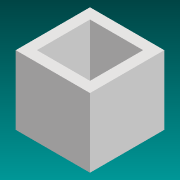
# Autodesk Inventor part: 龙门架柱1
Saved by Autodesk Inventor 2021 (Build 250183000, 183)
## iProperties
Created: 2025-04-17
Part Number: 龙门架柱1
Material: 常规
Document SubType Name: Modeling
Designer: 86155
Density: 1 g/cm^3
Appearance: 默认
Author: 86155
Autodesk Inventor part; units mm, degrees
ref_plane "YZ Plane" through (0, 0, 0) normal (1, 0, 0) x (0, 1, 0)
ref_plane "XY Plane" through (0, 0, 0) normal (0, 0, 1) x (1, 0, 0)
sketch "草图1" plane through (0, 0, 0) normal (0, 1, 0) x (-1, 0, 0)
  line L0 (0, 0) -> (-70, 0)
  line L1 (-70, 0) -> (-70, -70)
  line L2 (-70, -70) -> (0, -70)
  line L3 (0, -70) -> (0, 0)
  dimension "d0" = 70
  dimension "d1" = 70
  constraints: 8 end point, 2 parallel, 1 horizontal, 1 perpendicular
  measures "d0" distance of L2.end L1.end
  measures "d1" distance of L1.end L0.end
extrude "拉伸1" add sketch "草图1" along normal blind 5
sketch "草图2" plane through (0, 5, 0) normal (0, 1, 0) x (1, 0, 0)
  line L0 (0, 70) -> (0, 0) projected
  line L1 (70, 70) -> (0, 70) projected
  line L2 (0, 0) -> (70, 0)
  line L3 (70, 0) -> (70, 70)
  line L4 (70, 70) -> (0, 70)
  line L5 (0, 70) -> (0, 0)
  line L6 (60, 60) -> (60, 10)
  line L7 (60, 10) -> (10, 10)
  line L8 (10, 10) -> (10, 60)
  line L9 (10, 60) -> (60, 60)
  dimension "d4" = 10
  constraints: 16 end point, 4 parallel, 2 perpendicular, 1 horizontal, 3 other
  measures "d4" distance between parallel lines of L3 L6
extrude "拉伸2" add sketch "草图2" along normal blind 60
fillet "圆角1" radius 5 8 edges at (0, 32.5, 0) (35, 0, 0) (0, 0, -35) (35, 0, -70) (70, 0, -35) (70, 32.5, -70) (70, 32.5, 0) (0, 32.5, -70)
sketch "草图3" plane through (0, 65, 0) normal (0, 1, 0) x (1, 0, 0)
  arc A0 (0, 5) -> (5, 0) centre (5, 5) ccw projected
  line L0 (5, 0) -> (65, 0) projected
  arc A1 (65, 0) -> (70, 5) centre (65, 5) ccw projected
  line L1 (70, 5) -> (70, 65) projected
  arc A2 (70, 65) -> (65, 70) centre (65, 65) ccw projected
  line L2 (65, 70) -> (5, 70) projected
  arc A3 (5, 70) -> (0, 65) centre (5, 65) ccw projected
  line L3 (0, 65) -> (0, 5) projected
  line L4 (60, 60) -> (60, 10) projected
  line L5 (60, 10) -> (10, 10) projected
  line L6 (10, 10) -> (10, 60) projected
  line L7 (10, 60) -> (60, 60) projected
  line L8 (68.5, 65) -> (68.5, 5)
  arc A4 (65, 1.5) -> (68.5, 5) centre (65, 5) ccw
  line L9 (65, 1.5) -> (5, 1.5)
  arc A5 (1.5, 5) -> (5, 1.5) centre (5, 5) ccw
  line L10 (1.5, 5) -> (1.5, 65)
  arc A6 (5, 68.5) -> (1.5, 65) centre (5, 65) ccw
  line L11 (5, 68.5) -> (65, 68.5)
  arc A7 (68.5, 65) -> (65, 68.5) centre (65, 65) ccw
  line L12 (1.5, 45) -> (0, 45)
  line L13 (0, 65) -> (0, 5) projected
  line L14 (1.5, 25) -> (0, 25)
  point P0 (0, 0)
  dimension "d8" = 1.5
  dimension "d9" = 25
  dimension "d10" = 25
  constraints: 12 end point, 8 point on circle, 4 centre point, 4 point on line, 2 perpendicular, 7 other
  measures "d8" distance between parallel lines of L1 L8
  measures "d9" distance between parallel lines of L2 L12
  measures "d10" distance between parallel lines of L0 L14
extrude "拉伸3" add sketch "草图3" along normal blind 450 contours L3 L14 L10 A5 L9 A4 L8 A7 L11 A6 L12 A3 L2 A2 L1 A1 L0 A0
ref_plane "工作平面1" through (0, 130, 0) normal (0, 1, 0) x (-1, 0, 0)
sketch "草图5" plane through (0, 130, 0) normal (0, 1, 0) x (-1, 0, 0)
  arc A0 (-70, -65) -> (-65, -70) centre (-65, -65) ccw projected
  line L0 (-65, -70) -> (-5, -70)
  line L1 (-5, -70) -> (-5, -80)
  line L2 (-5, -80) -> (-65, -80)
  line L3 (-65, -80) -> (-65, -70)
  point P0 (0, 0)
  dimension "d18" = 10
  constraints: 8 end point, 2 parallel, 1 horizontal, 1 perpendicular
  measures "d18" distance of L0.end L1.end
extrude "拉伸4" add sketch "草图5" along normal blind 10
fillet "圆角2" radius 10 2 edges at (65, 135, -80) (5, 135, -80)
sketch "草图6" plane through (0, 140, 0) normal (0, 1, 0) x (1, 0, 0)
  point P0 (0, 0)
sketch "草图7" plane through (0, 140, 0) normal (0, 1, 0) x (1, 0, 0)
  arc A0 (65, 70) -> (55, 80) centre (55, 70) ccw projected
  line L0 (55, 80) -> (15, 80) projected
  arc A1 (15, 80) -> (5, 70) centre (15, 70) ccw projected
  arc A2 (62.5, 70) -> (55, 77.5) centre (55, 70) ccw
  line L1 (55, 77.5) -> (15, 77.5)
  arc A3 (15, 77.5) -> (7.5, 70) centre (15, 70) ccw
  line L2 (62.5, 70) -> (7.5, 70)
  line L3 (60, 10) -> (60, 60) projected
  point P0 (0, 0)
  dimension "d22" = 2.5
  constraints: 4 end point, 4 point on circle, 2 centre point, 1 perpendicular, 2 other
  measures "d22" radial gap between concentric circles of A0 A2
extrude "拉伸5" cut sketch "草图7" against normal blind 2
ref_plane "工作平面2" through (0, 485, 0) normal (0, 1, 0) x (1, 0, 0)
sketch "草图8" plane through (0, 485, 0) normal (0, 1, 0) x (1, 0, 0)
  arc A0 (15, 80) -> (5, 70) centre (15, 70) ccw projected
  line L0 (55, 80) -> (15, 80) projected
  arc A1 (65, 70) -> (55, 80) centre (55, 70) ccw projected
  line L1 (5, 70) -> (65, 70) projected
  point P0 (0, 0)
extrude "拉伸6" add sketch "草图8" along normal blind 10
sketch "草图9" plane through (0, 485, 0) normal (0, -1, 0) x (1, 0, 0)
  line L0 (15, -77.5) -> (55, -77.5) projected
  arc A0 (7.5, -70) -> (15, -77.5) centre (15, -70) ccw projected
  line L1 (62.5, -70) -> (7.5, -70) projected
  arc A1 (55, -77.5) -> (62.5, -70) centre (55, -70) ccw projected
  point P0 (0, 0)
extrude "拉伸7" cut sketch "草图9" against normal blind 2
